Autodesk Fusion 360 part; units mm, degrees
(part 2 of 2)
  line L920 (94.2802, 13.415) -> (94.312, 13.3328)
  line L921 (90.8458, 12.0108) -> (90.0144, 12.5127)
  line L922 (98.4562, 13.1514) -> (98.2574, 14.132)
  line L923 (107.9148, 10.617) -> (107.3286, 10.4149)
  line L924 (98.2574, 14.132) -> (98.2624, 14.3913)
  line L925 (86.8526, 11.9567) -> (86.9805, 11.3055)
  line L926 (105.7225, 13.415) -> (105.8246, 13.9347)
  line L927 (107.3286, 10.4149) -> (105.3566, 11.5535)
  line L928 (94.1781, 13.9347) -> (94.2802, 13.415)
  line L929 (91.4254, 11.3668) -> (91.3001, 11.5939)
  line L930 (88.0455, 13.1497) -> (87.3969, 12.6054)
  line L931 (87.4895, 9.9878) -> (87.9914, 9.1564)
  line L932 (97.6083, 15.8299) -> (96.7216, 16.9295)
  line L933 (108.5772, 11.3668) -> (107.9148, 10.617)
  line L934 (94.6461, 11.5535) -> (92.674, 10.4149)
  line L935 (105.3566, 11.5535) -> (105.2385, 12.1621)
  line L936 (87.9914, 9.1564) -> (88.3397, 8.7574)
  line L937 (88.3397, 8.7574) -> (88.4083, 8.702)
  line L938 (102.3944, 15.8299) -> (101.9253, 14.9795)
  line L939 (105.2385, 12.1621) -> (105.5566, 13.1108)
  line L940 (105.5566, 13.1108) -> (105.6907, 13.3328)
  line L941 (103.781, 17.3659) -> (103.2811, 16.9295)
  line L942 (90.0144, 12.5127) -> (88.6967, 13.0217)
  line L943 (86.9805, 11.3055) -> (87.4895, 9.9878)
  line L944 (95.3877, 17.2189) -> (94.592, 16.9293)
  line L945 (108.7578, 11.6625) -> (108.7025, 11.5939)
  line L946 (87.3969, 12.6054) -> (86.8526, 11.9567)
  line L947 (101.9253, 14.9795) -> (101.7539, 14.4784)
  line L948 (101.5465, 13.1514) -> (101.1399, 12.6833)
  line L949 (94.592, 16.9293) -> (94.3773, 16.3014)
  line L950 (103.2811, 16.9295) -> (102.3944, 15.8299)
  line L951 (105.8246, 13.9347) -> (105.8435, 14.9057)
  line L952 (101.1399, 12.6833) -> (98.8628, 12.6833)
  line L953 (94.3773, 16.3014) -> (94.1592, 14.9057)
  line L954 (96.2216, 17.3659) -> (95.3877, 17.2189)
  line L955 (94.1592, 14.9057) -> (94.1781, 13.9347)
  line L956 (108.7025, 11.5939) -> (108.5772, 11.3668)
  line L957 (94.7641, 12.1621) -> (94.6461, 11.5535)
  line L958 (94.446, 13.1108) -> (94.7641, 12.1621)
  line L959 (92.0879, 10.617) -> (91.4254, 11.3668)
  line L960 (96.7216, 16.9295) -> (96.2216, 17.3659)
  line L961 (94.312, 13.3328) -> (94.446, 13.1108)
  line L962 (87.84, 5.238) -> (86.8914, 5.5562)
  line L963 (89.3852, 7.9143) -> (89.5873, 7.3281)
  line L964 (101.7403, 14.3913) -> (101.7453, 14.132)
  line L965 (86.6694, 5.6902) -> (86.5872, 5.7219)
  line L966 (109.9882, 12.5127) -> (109.1568, 12.0108)
  line L967 (86.8914, 5.5562) -> (86.6694, 5.6902)
  line L968 (98.8628, 12.6833) -> (98.4562, 13.1514)
  line L969 (91.3001, 11.5939) -> (91.2448, 11.6625)
  line L970 (104.6149, 17.2189) -> (103.781, 17.3659)
  line L971 (105.4106, 16.9293) -> (104.6149, 17.2189)
  line L972 (105.6254, 16.3014) -> (105.4106, 16.9293)
  line L973 (88.4083, 8.702) -> (88.6354, 8.5768)
  line L974 (88.6354, 8.5768) -> (89.3852, 7.9143)
  line L975 (101.7539, 14.4784) -> (101.7403, 14.3913)
  line L976 (89.5873, 7.3281) -> (88.4487, 5.3561)
  line L977 (86.5872, 5.7219) -> (86.0675, 5.8241)
  line L978 (85.0965, 5.8431) -> (83.7008, 5.625)
  line L979 (88.4487, 5.3561) -> (87.84, 5.238)
  line L980 (86.0675, 5.8241) -> (85.0965, 5.8431)
  line L981 (83.7008, 5.625) -> (83.0729, 5.4103)
  line L982 (83.0729, -5.4081) -> (83.7008, -5.6228)
  line L983 (87.3189, 1.1396) -> (87.3189, -1.1375)
  line L984 (82.6363, -3.7785) -> (82.7833, -4.6124)
  line L985 (85.8702, 1.745) -> (86.8508, 1.5462)
  line L986 (83.0727, -3.2785) -> (82.6363, -3.7785)
  line L987 (86.6694, -5.688) -> (86.8914, -5.554)
  line L988 (82.7833, 4.6146) -> (82.6363, 3.7807)
  line L989 (82.6363, 3.7807) -> (83.0727, 3.2807)
  line L990 (85.0227, 1.925) -> (85.5238, 1.7535)
  line L991 (86.8914, -5.554) -> (87.84, -5.2359)
  line L992 (85.5238, 1.7535) -> (85.6109, 1.74)
  line L993 (84.1723, 2.394) -> (85.0227, 1.925)
  line L994 (85.5238, -1.7513) -> (85.0227, -1.9227)
  line L995 (85.0227, -1.9227) -> (84.1723, -2.3918)
  line L996 (85.6109, -1.7379) -> (85.5238, -1.7513)
  line L997 (105.6254, -16.2992) -> (105.8435, -14.9035)
  line L998 (94.3773, -16.2992) -> (94.592, -16.9271)
  line L999 (83.0727, 3.2807) -> (84.1723, 2.394)
  line L1000 (88.4487, -5.3539) -> (89.5873, -7.326)
  line L1001 (85.0965, -5.841) -> (86.0675, -5.8219)
  line L1002 (88.3397, -8.7552) -> (87.9914, -9.1542)
  line L1003 (95.3877, -17.2167) -> (96.2216, -17.3637)
  line L1004 (84.1723, -2.3918) -> (83.0727, -3.2785)
  line L1005 (82.7833, -4.6124) -> (83.0729, -5.4081)
  line L1006 (85.6109, 1.74) -> (85.8702, 1.745)
  line L1007 (86.0675, -5.8219) -> (86.5872, -5.7198)
  line L1008 (86.8508, -1.5441) -> (85.8702, -1.7429)
  line L1009 (86.5872, -5.7198) -> (86.6694, -5.688)
  line L1010 (86.8508, 1.5462) -> (87.3189, 1.1396)
  line L1011 (83.0729, 5.4103) -> (82.7833, 4.6146)
  line L1012 (87.3189, -1.1375) -> (86.8508, -1.5441)
  line L1013 (83.7008, -5.6228) -> (85.0965, -5.841)
  line L1014 (105.8435, -14.9035) -> (105.8246, -13.9325)
  line L1015 (98.2624, -14.3891) -> (98.2574, -14.1298)
  line L1016 (105.5566, -13.1086) -> (105.2385, -12.16)
  line L1017 (104.6149, -17.2167) -> (105.4106, -16.9271)
  line L1018 (90.0144, -12.5106) -> (90.8458, -12.0087)
  line L1019 (105.2385, -12.16) -> (105.3566, -11.5513)
  line L1020 (85.8702, -1.7429) -> (85.6109, -1.7379)
  line L1021 (105.8246, -13.9325) -> (105.7225, -13.4128)
  line L1022 (94.7641, -12.16) -> (94.446, -13.1086)
  line L1023 (101.5465, -13.1492) -> (101.7453, -14.1298)
  line L1024 (105.6907, -13.3306) -> (105.5566, -13.1086)
  line L1025 (89.3852, -7.9121) -> (88.6354, -8.5746)
  line L1026 (88.4083, -8.6999) -> (88.3397, -8.7552)
  line L1027 (94.2802, -13.4128) -> (94.1781, -13.9325)
  line L1028 (101.7403, -14.3891) -> (101.7539, -14.4762)
  line L1029 (105.7225, -13.4128) -> (105.6907, -13.3306)
  line L1030 (90.8458, -12.0087) -> (91.2448, -11.6604)
  line L1031 (89.5873, -7.326) -> (89.3852, -7.9121)
  line L1032 (88.0455, -13.1475) -> (88.6967, -13.0195)
  line L1033 (88.6967, -13.0195) -> (90.0144, -12.5106)
  line L1034 (103.2811, -16.9273) -> (103.781, -17.3637)
  line L1035 (92.674, -10.4128) -> (94.6461, -11.5513)
  line L1036 (107.9148, -10.6149) -> (108.5772, -11.3647)
  line L1037 (94.1781, -13.9325) -> (94.1592, -14.9035)
  line L1038 (96.2216, -17.3637) -> (96.7216, -16.9273)
  line L1039 (88.6354, -8.5746) -> (88.4083, -8.6999)
  line L1040 (94.592, -16.9271) -> (95.3877, -17.2167)
  line L1041 (94.312, -13.3306) -> (94.2802, -13.4128)
  line L1042 (98.2488, -14.4762) -> (98.2624, -14.3891)
  line L1043 (103.781, -17.3637) -> (104.6149, -17.2167)
  line L1044 (87.84, -5.2359) -> (88.4487, -5.3539)
  line L1045 (94.446, -13.1086) -> (94.312, -13.3306)
  line L1046 (101.7539, -14.4762) -> (101.9253, -14.9773)
  line L1047 (113.0221, 11.3055) -> (113.1501, 11.9567)
  line L1048 (98.4562, -13.1492) -> (98.8628, -12.6811)
  line L1049 (111.6629, -8.7552) -> (111.5943, -8.6999)
  line L1050 (98.2574, -14.1298) -> (98.4562, -13.1492)
  line L1051 (94.6461, -11.5513) -> (94.7641, -12.16)
  line L1052 (92.0879, -10.6149) -> (92.674, -10.4128)
  line L1053 (111.9571, -13.1475) -> (112.6058, -12.6032)
  line L1054 (91.4254, -11.3647) -> (92.0879, -10.6149)
  line L1055 (98.8628, -12.6811) -> (101.1399, -12.6811)
  line L1056 (91.3001, -11.5917) -> (91.4254, -11.3647)
  line L1057 (87.4895, -9.9856) -> (86.9805, -11.3034)
  line L1058 (105.4106, -16.9271) -> (105.6254, -16.2992)
  line L1059 (87.3969, -12.6032) -> (88.0455, -13.1475)
  line L1060 (86.9805, -11.3034) -> (86.8526, -11.9545)
  line L1061 (108.7025, -11.5917) -> (108.7578, -11.6604)
  line L1062 (105.3566, -11.5513) -> (107.3286, -10.4128)
  line L1063 (107.3286, -10.4128) -> (107.9148, -10.6149)
  line L1064 (110.6175, -7.9121) -> (110.4154, -7.326)
  line L1065 (98.0774, -14.9773) -> (98.2488, -14.4762)
  line L1066 (115.8303, -2.3918) -> (114.9799, -1.9227)
  line L1067 (87.9914, -9.1542) -> (87.4895, -9.9856)
  line L1068 (114.3917, 1.74) -> (114.4788, 1.7535)
  line L1069 (94.1592, -14.9035) -> (94.3773, -16.2992)
  line L1070 (116.3018, -5.6228) -> (116.9297, -5.4081)
  line L1071 (116.9299, 3.2807) -> (117.3664, 3.7807)
  line L1072 (102.3944, -15.8277) -> (103.2811, -16.9273)
  line L1073 (97.6083, -15.8277) -> (98.0774, -14.9773)
  line L1074 (101.1399, -12.6811) -> (101.5465, -13.1492)
  line L1075 (114.9061, -5.841) -> (116.3018, -5.6228)
  line L1076 (111.5943, -8.6999) -> (111.3673, -8.5746)
  line L1077 (101.9253, -14.9773) -> (102.3944, -15.8277)
  line L1078 (108.5772, -11.3647) -> (108.7025, -11.5917)
  line L1079 (91.2448, -11.6604) -> (91.3001, -11.5917)
  line L1080 (101.7453, -14.1298) -> (101.7403, -14.3891)
  line L1081 (86.8526, -11.9545) -> (87.3969, -12.6032)
  line L1082 (112.1626, 5.238) -> (111.5539, 5.3561)
  line L1083 (116.3018, 5.625) -> (114.9061, 5.8431)
  line L1084 (112.0112, 9.1564) -> (112.5131, 9.9878)
  line L1085 (108.7578, -11.6604) -> (109.1568, -12.0087)
  line L1086 (114.9061, 5.8431) -> (113.9351, 5.8241)
  line L1087 (111.306, -13.0195) -> (111.9571, -13.1475)
  line L1088 (96.7216, -16.9273) -> (97.6083, -15.8277)
  line L1089 (109.1568, 12.0108) -> (108.7578, 11.6625)
  line L1090 (114.4788, -1.7513) -> (114.3917, -1.7379)
  line L1091 (111.5539, 5.3561) -> (110.4154, 7.3281)
  line L1092 (113.1501, 11.9567) -> (112.6058, 12.6054)
  line L1093 (112.6837, -1.1375) -> (112.6837, 1.1396)
  line L1094 (115.8303, 2.394) -> (116.9299, 3.2807)
  line L1095 (110.6175, 7.9143) -> (111.3673, 8.5768)
  line L1096 (113.4154, 5.7219) -> (113.3332, 5.6902)
  line L1097 (112.5131, 9.9878) -> (113.0221, 11.3055)
  line L1098 (113.4154, -5.7198) -> (113.9351, -5.8219)
  line L1099 (112.6058, 12.6054) -> (111.9571, 13.1497)
  line L1100 (114.1324, -1.7429) -> (113.1518, -1.5441)
  line L1101 (110.4154, 7.3281) -> (110.6175, 7.9143)
  line L1102 (113.1518, 1.5462) -> (114.1324, 1.745)
  line L1103 (110.4154, -7.326) -> (111.5539, -5.3539)
  line L1104 (114.4788, 1.7535) -> (114.9799, 1.925)
  line L1105 (112.6058, -12.6032) -> (113.1501, -11.9545)
  line L1106 (113.1501, -11.9545) -> (113.0221, -11.3034)
  line L1107 (113.1112, 5.5562) -> (112.1626, 5.238)
  line L1108 (113.0221, -11.3034) -> (112.5131, -9.9856)
  line L1109 (109.1568, -12.0087) -> (109.9882, -12.5106)
  line L1110 (111.6629, 8.7574) -> (112.0112, 9.1564)
  line L1111 (114.1324, 1.745) -> (114.3917, 1.74)
  line L1112 (111.3673, -8.5746) -> (110.6175, -7.9121)
  line L1113 (111.306, 13.0217) -> (109.9882, 12.5127)
  line L1114 (112.1626, -5.2359) -> (113.1112, -5.554)
  line L1115 (117.3664, -3.7785) -> (116.9299, -3.2785)
  line L1116 (116.9297, 5.4103) -> (116.3018, 5.625)
  line L1117 (113.9351, -5.8219) -> (114.9061, -5.841)
  line L1118 (113.1112, -5.554) -> (113.3332, -5.688)
  line L1119 (111.3673, 8.5768) -> (111.5943, 8.702)
  line L1120 (117.2193, -4.6124) -> (117.3664, -3.7785)
  line L1121 (113.3332, -5.688) -> (113.4154, -5.7198)
  line L1122 (109.9882, -12.5106) -> (111.306, -13.0195)
  line L1123 (113.9351, 5.8241) -> (113.4154, 5.7219)
  line L1124 (116.9297, -5.4081) -> (117.2193, -4.6124)
  line L1125 (114.3917, -1.7379) -> (114.1324, -1.7429)
  line L1126 (111.5539, -5.3539) -> (112.1626, -5.2359)
  line L1127 (113.1518, -1.5441) -> (112.6837, -1.1375)
  line L1128 (113.3332, 5.6902) -> (113.1112, 5.5562)
  line L1129 (112.5131, -9.9856) -> (112.0112, -9.1542)
  line L1130 (116.9299, -3.2785) -> (115.8303, -2.3918)
  line L1131 (111.9571, 13.1497) -> (111.306, 13.0217)
  line L1132 (117.2193, 4.6146) -> (116.9297, 5.4103)
  line L1133 (117.3664, 3.7807) -> (117.2193, 4.6146)
  line L1134 (114.9799, -1.9227) -> (114.4788, -1.7513)
  line L1135 (92.674, 10.4149) -> (92.0879, 10.617)
  line L1136 (98.2488, 14.4784) -> (98.0774, 14.9795)
  line L1137 (111.5943, 8.702) -> (111.6629, 8.7574)
  line L1138 (114.9799, 1.925) -> (115.8303, 2.394)
  line L1139 (112.6837, 1.1396) -> (113.1518, 1.5462)
  line L1140 (112.0112, -9.1542) -> (111.6629, -8.7552)
  circle A0 centre (0, 0) radius 4
  line L1141 (102.5, 5) -> (97.5, 5)
  line L1142 (97.5, 5) -> (97.5, -5)
  line L1143 (97.5, -5) -> (102.5, -5)
  line L1144 (102.5, -5) -> (102.5, 5)
  line L1145 (102.5, 5) -> (97.5, -5) construction
  line L1146 (97.5, 5) -> (102.5, -5) construction
  arc A1 (11.1765, 46.1664) -> (5, 41.3068) centre (10, 41.3068) ccw
  arc A2 (-5, 41.3068) -> (-11.1765, 46.1664) centre (-10, 41.3068) ccw
  arc A3 (-46.1664, 11.1765) -> (-41.3068, 5) centre (-41.3068, 10) ccw
  arc A4 (-41.3068, -5) -> (-46.1664, -11.1765) centre (-41.3068, -10) ccw
  arc A5 (-11.1765, -46.1664) -> (-5, -41.3068) centre (-10, -41.3068) ccw
  arc A6 (5, -41.3068) -> (11.1765, -46.1664) centre (10, -41.3068) ccw
  arc A7 (46.1664, -11.1765) -> (41.3068, -5) centre (41.3068, -10) ccw
  arc A8 (41.3068, 5) -> (46.1664, 11.1765) centre (41.3068, 10) ccw
  arc A9 (-11.1765, 46.1664) -> (-46.1664, 11.1765) centre (0, 0) ccw
  arc A10 (46.1664, 11.1765) -> (11.1765, 46.1664) centre (0, 0) ccw
  arc A11 (-46.1664, -11.1765) -> (-11.1765, -46.1664) centre (0, 0) ccw
  arc A12 (11.1765, -46.1664) -> (46.1664, -11.1765) centre (0, 0) ccw
  arc A13 (-18.3303, -5) -> (-5, -18.3303) centre (0, 0) ccw
  arc A14 (5, -18.3303) -> (18.3303, -5) centre (0, 0) ccw
  arc A15 (18.3303, 5) -> (5, 18.3303) centre (0, 0) ccw
  arc A16 (-5, 18.3303) -> (-18.3303, 5) centre (0, 0) ccw
  line L1147 (-5, 41.3068) -> (-5, 18.3303)
  line L1148 (-5, -18.3303) -> (-5, -41.3068)
  line L1149 (5, -41.3068) -> (5, -18.3303)
  line L1150 (5, 18.3303) -> (5, 41.3068)
  line L1151 (18.3303, 5) -> (41.3068, 5)
  line L1152 (41.3068, -5) -> (18.3303, -5)
  line L1153 (-18.3303, -5) -> (-41.3068, -5)
  line L1154 (-41.3068, 5) -> (-18.3303, 5)
  line L1155 (133.0727, 3.2807) -> (134.1723, 2.394)
  line L1156 (135.0227, 1.925) -> (135.5238, 1.7535)
  line L1157 (139.5873, 7.3281) -> (138.4487, 5.3561)
  line L1158 (136.6694, 5.6902) -> (136.5872, 5.7219)
  line L1159 (137.3969, 12.6054) -> (136.8526, 11.9567)
  line L1160 (148.4562, 13.1514) -> (148.2574, 14.132)
  line L1161 (138.0455, 13.1497) -> (137.3969, 12.6054)
  line L1162 (135.8702, 1.745) -> (136.8508, 1.5462)
  line L1163 (138.3397, 8.7574) -> (138.4083, 8.702)
  line L1164 (134.1723, 2.394) -> (135.0227, 1.925)
  line L1165 (136.8508, 1.5462) -> (137.3189, 1.1396)
  line L1166 (132.7833, 4.6146) -> (132.6363, 3.7807)
  line L1167 (138.6967, 13.0217) -> (138.0455, 13.1497)
  line L1168 (148.0774, 14.9795) -> (147.6083, 15.8299)
  line L1169 (138.4487, 5.3561) -> (137.84, 5.238)
  line L1170 (132.6363, 3.7807) -> (133.0727, 3.2807)
  line L1171 (138.6354, 8.5768) -> (139.3852, 7.9143)
  line L1172 (136.8526, 11.9567) -> (136.9805, 11.3055)
  line L1173 (136.8914, 5.5562) -> (136.6694, 5.6902)
  line L1174 (137.9914, 9.1564) -> (138.3397, 8.7574)
  line L1175 (136.9805, 11.3055) -> (137.4895, 9.9878)
  line L1176 (137.4895, 9.9878) -> (137.9914, 9.1564)
  line L1177 (133.0729, 5.4103) -> (132.7833, 4.6146)
  line L1178 (136.5872, 5.7219) -> (136.0675, 5.8241)
  line L1179 (135.6109, 1.74) -> (135.8702, 1.745)
  line L1180 (136.0675, 5.8241) -> (135.0965, 5.8431)
  line L1181 (137.84, 5.238) -> (136.8914, 5.5562)
  line L1182 (139.3852, 7.9143) -> (139.5873, 7.3281)
  line L1183 (135.5238, 1.7535) -> (135.6109, 1.74)
  line L1184 (133.7008, 5.625) -> (133.0729, 5.4103)
  line L1185 (135.0965, 5.8431) -> (133.7008, 5.625)
  line L1186 (138.4083, 8.702) -> (138.6354, 8.5768)
  line L1187 (140.0144, 12.5127) -> (138.6967, 13.0217)
  line L1188 (137.3189, 1.1396) -> (137.3189, -1.1375)
  line L1189 (151.5465, -13.1492) -> (151.7453, -14.1298)
  line L1190 (154.6149, -17.2167) -> (155.4106, -16.9271)
  line L1191 (151.9253, -14.9773) -> (152.3944, -15.8277)
  line L1192 (162.6058, -12.6032) -> (163.1501, -11.9545)
  line L1193 (158.7578, -11.6604) -> (159.1568, -12.0087)
  line L1194 (155.2385, -12.16) -> (155.3566, -11.5513)
  line L1195 (155.6254, -16.2992) -> (155.8435, -14.9035)
  line L1196 (158.5772, -11.3647) -> (158.7025, -11.5917)
  line L1197 (155.7225, -13.4128) -> (155.6907, -13.3306)
  line L1198 (159.1568, -12.0087) -> (159.9882, -12.5106)
  line L1199 (152.3944, -15.8277) -> (153.2811, -16.9273)
  line L1200 (158.7025, -11.5917) -> (158.7578, -11.6604)
  line L1201 (161.9571, -13.1475) -> (162.6058, -12.6032)
  line L1202 (161.306, -13.0195) -> (161.9571, -13.1475)
  line L1203 (167.3664, -3.7785) -> (166.9299, -3.2785)
  line L1204 (161.3673, -8.5746) -> (160.6175, -7.9121)
  line L1205 (151.7403, -14.3891) -> (151.7539, -14.4762)
  line L1206 (164.3917, -1.7379) -> (164.1324, -1.7429)
  line L1207 (163.1112, -5.554) -> (163.3332, -5.688)
  line L1208 (161.5943, -8.6999) -> (161.3673, -8.5746)
  line L1209 (155.5566, -13.1086) -> (155.2385, -12.16)
  line L1210 (165.8303, -2.3918) -> (164.9799, -1.9227)
  line L1211 (162.5131, -9.9856) -> (162.0112, -9.1542)
  line L1212 (151.1399, -12.6811) -> (151.5465, -13.1492)
  line L1213 (161.5539, -5.3539) -> (162.1626, -5.2359)
  line L1214 (166.9299, -3.2785) -> (165.8303, -2.3918)
  line L1215 (163.3332, -5.688) -> (163.4154, -5.7198)
  line L1216 (167.2193, -4.6124) -> (167.3663, -3.7785)
  line L1217 (157.9148, -10.6149) -> (158.5772, -11.3647)
  line L1218 (164.1324, -1.7429) -> (163.1518, -1.5441)
  line L1219 (163.9351, -5.8219) -> (164.9061, -5.841)
  line L1220 (166.3018, -5.6228) -> (166.9297, -5.4081)
  line L1221 (164.9799, -1.9227) -> (164.4788, -1.7513)
  line L1222 (162.1626, -5.2359) -> (163.1112, -5.554)
  line L1223 (160.4154, -7.326) -> (161.5539, -5.3539)
  line L1224 (166.9297, -5.4081) -> (167.2193, -4.6124)
  line L1225 (162.0112, -9.1542) -> (161.6629, -8.7552)
  line L1226 (163.4154, -5.7198) -> (163.9351, -5.8219)
  line L1227 (160.6175, -7.9121) -> (160.4154, -7.326)
  line L1228 (163.1518, -1.5441) -> (162.6837, -1.1375)
  line L1229 (164.4788, -1.7513) -> (164.3917, -1.7379)
  line L1230 (164.9061, -5.841) -> (166.3018, -5.6228)
  line L1231 (161.6629, -8.7552) -> (161.5943, -8.6999)
  line L1232 (161.5943, 8.702) -> (161.6629, 8.7574)
  line L1233 (166.9297, 5.4103) -> (166.3018, 5.625)
  line L1234 (164.4788, 1.7535) -> (164.9799, 1.925)
  line L1235 (163.1518, 1.5462) -> (164.1324, 1.745)
  line L1236 (164.9799, 1.925) -> (165.8303, 2.394)
  line L1237 (163.0221, -11.3034) -> (162.5131, -9.9856)
  line L1238 (161.6629, 8.7574) -> (162.0112, 9.1564)
  line L1239 (167.3664, 3.7807) -> (167.2193, 4.6146)
  line L1240 (162.0112, 9.1564) -> (162.5131, 9.9878)
  line L1241 (166.9299, 3.2807) -> (167.3663, 3.7807)
  line L1242 (167.2193, 4.6146) -> (166.9297, 5.4103)
  line L1243 (160.4154, 7.3281) -> (160.6175, 7.9143)
  line L1244 (164.9061, 5.8431) -> (163.9351, 5.8241)
  line L1245 (161.5539, 5.3561) -> (160.4154, 7.3281)
  line L1246 (151.7453, 14.132) -> (151.5465, 13.1514)
  line L1247 (163.0221, 11.3055) -> (163.1501, 11.9567)
  line L1248 (162.1626, 5.238) -> (161.5539, 5.3561)
  line L1249 (161.9571, 13.1497) -> (161.306, 13.0217)
  line L1250 (155.8435, 14.9057) -> (155.6254, 16.3014)
  line L1251 (151.7539, 14.4784) -> (151.7403, 14.3913)
  line L1252 (161.3673, 8.5768) -> (161.5943, 8.702)
  line L1253 (159.1568, 12.0108) -> (158.7578, 11.6625)
  line L1254 (151.5465, 13.1514) -> (151.1399, 12.6833)
  line L1255 (158.7578, 11.6625) -> (158.7025, 11.5939)
  line L1256 (155.4106, 16.9293) -> (154.6149, 17.2189)
  line L1257 (155.8246, 13.9347) -> (155.8435, 14.9057)
  line L1258 (160.6175, 7.9143) -> (161.3673, 8.5768)
  line L1259 (166.3018, 5.625) -> (164.9061, 5.8431)
  line L1260 (164.1324, 1.745) -> (164.3917, 1.74)
  line L1261 (162.5131, 9.9878) -> (163.0221, 11.3055)
  line L1262 (162.6058, 12.6054) -> (161.9571, 13.1497)
  line L1263 (155.6254, 16.3014) -> (155.4106, 16.9293)
  line L1264 (163.1112, 5.5562) -> (162.1626, 5.238)
  line L1265 (163.1501, 11.9567) -> (162.6058, 12.6054)
  line L1266 (152.3944, 15.8299) -> (151.9253, 14.9795)
  line L1267 (151.7403, 14.3913) -> (151.7453, 14.132)
  line L1268 (165.8303, 2.394) -> (166.9299, 3.2807)
  line L1269 (162.6837, 1.1396) -> (163.1518, 1.5462)
  line L1270 (164.3917, 1.74) -> (164.4788, 1.7535)
  line L1271 (163.3332, 5.6902) -> (163.1112, 5.5562)
  line L1272 (163.9351, 5.8241) -> (163.4154, 5.7219)
  line L1273 (163.4154, 5.7219) -> (163.3332, 5.6902)
  line L1274 (155.7225, 13.415) -> (155.8246, 13.9347)
  line L1275 (151.9253, 14.9795) -> (151.7539, 14.4784)
  line L1276 (147.6083, -15.8277) -> (148.0774, -14.9773)
  line L1277 (157.3286, 10.4149) -> (155.3566, 11.5535)
  line L1278 (155.2385, 12.1621) -> (155.5566, 13.1108)
  line L1279 (148.2488, -14.4762) -> (148.2624, -14.3891)
  line L1280 (144.592, -16.9271) -> (145.3877, -17.2167)
  line L1281 (144.7641, -12.16) -> (144.446, -13.1086)
  line L1282 (162.6837, -1.1375) -> (162.6837, 1.1396)
  line L1283 (153.2811, 16.9295) -> (152.3944, 15.8299)
  line L1284 (148.2574, -14.1298) -> (148.4562, -13.1492)
  line L1285 (155.3566, 11.5535) -> (155.2385, 12.1621)
  line L1286 (140.8458, -12.0087) -> (141.2448, -11.6604)
  line L1287 (142.674, -10.4128) -> (144.6461, -11.5513)
  line L1288 (146.7216, -16.9273) -> (147.6083, -15.8277)
  line L1289 (141.2448, -11.6604) -> (141.3001, -11.5917)
  line L1290 (158.5772, 11.3668) -> (157.9148, 10.617)
  line L1291 (154.6149, 17.2189) -> (153.781, 17.3659)
  line L1292 (161.306, 13.0217) -> (159.9882, 12.5127)
  line L1293 (144.1592, -14.9035) -> (144.3773, -16.2992)
  line L1294 (157.9148, 10.617) -> (157.3286, 10.4149)
  line L1295 (148.0774, -14.9773) -> (148.2488, -14.4762)
  line L1296 (141.3001, -11.5917) -> (141.4254, -11.3647)
  line L1297 (155.5566, 13.1108) -> (155.6907, 13.3328)
  line L1298 (158.7025, 11.5939) -> (158.5772, 11.3668)
  line L1299 (141.4254, -11.3647) -> (142.0879, -10.6149)
  line L1300 (153.781, 17.3659) -> (153.2811, 16.9295)
  line L1301 (142.0879, -10.6149) -> (142.674, -10.4128)
  line L1302 (159.9882, 12.5127) -> (159.1568, 12.0108)
  line L1303 (155.6907, 13.3328) -> (155.7225, 13.415)
  line L1304 (144.1781, -13.9325) -> (144.1592, -14.9035)
  line L1305 (140.0144, -12.5106) -> (140.8458, -12.0087)
  line L1306 (148.4562, -13.1492) -> (148.8628, -12.6811)
  line L1307 (144.312, -13.3306) -> (144.2802, -13.4128)
  line L1308 (144.2802, -13.4128) -> (144.1781, -13.9325)
  line L1309 (137.3189, -1.1375) -> (136.8508, -1.5441)
  line L1310 (134.1723, -2.3918) -> (133.0727, -3.2785)
  line L1311 (137.9914, -9.1542) -> (137.4895, -9.9856)
  line L1312 (135.0965, -5.841) -> (136.0675, -5.8219)
  line L1313 (136.8914, -5.554) -> (137.84, -5.2359)
  line L1314 (148.2624, -14.3891) -> (148.2574, -14.1298)
  line L1315 (138.3397, -8.7552) -> (137.9914, -9.1542)
  line L1316 (133.0729, -5.4081) -> (133.7008, -5.6228)
  line L1317 (137.3969, -12.6032) -> (138.0455, -13.1475)
  line L1318 (138.0455, -13.1475) -> (138.6967, -13.0195)
  line L1319 (144.446, -13.1086) -> (144.312, -13.3306)
  line L1320 (136.0675, -5.8219) -> (136.5872, -5.7198)
  line L1321 (138.6354, -8.5746) -> (138.4083, -8.6999)
  line L1322 (151.1399, 12.6833) -> (148.8628, 12.6833)
  line L1323 (144.3773, -16.2992) -> (144.592, -16.9271)
  line L1324 (138.4083, -8.6999) -> (138.3397, -8.7552)
  line L1325 (136.8526, -11.9545) -> (137.3969, -12.6032)
  line L1326 (144.6461, -11.5513) -> (144.7641, -12.16)
  line L1327 (136.9805, -11.3034) -> (136.8526, -11.9545)
  line L1328 (135.0227, -1.9227) -> (134.1723, -2.3918)
  line L1329 (136.5872, -5.7198) -> (136.6694, -5.688)
  line L1330 (139.5873, -7.326) -> (139.3852, -7.9121)
  line L1331 (139.3852, -7.9121) -> (138.6354, -8.5746)
  line L1332 (138.4487, -5.3539) -> (139.5873, -7.326)
  line L1333 (132.6363, -3.7785) -> (132.7833, -4.6124)
  line L1334 (133.0727, -3.2785) -> (132.6363, -3.7785)
  line L1335 (132.7833, -4.6124) -> (133.0729, -5.4081)
  line L1336 (146.2216, -17.3637) -> (146.7216, -16.9273)
  line L1337 (145.3877, -17.2167) -> (146.2216, -17.3637)
  line L1338 (137.4895, -9.9856) -> (136.9805, -11.3034)
  line L1339 (137.84, -5.2359) -> (138.4487, -5.3539)
  line L1340 (135.6109, -1.7379) -> (135.5238, -1.7513)
  line L1341 (135.5238, -1.7513) -> (135.0227, -1.9227)
  line L1342 (148.8628, -12.6811) -> (151.1399, -12.6811)
  line L1343 (147.6083, 15.8299) -> (146.7216, 16.9295)
  line L1344 (136.6694, -5.688) -> (136.8914, -5.554)
  line L1345 (144.592, 16.9293) -> (144.3773, 16.3014)
  line L1346 (148.2488, 14.4784) -> (148.0774, 14.9795)
  line L1347 (148.2624, 14.3913) -> (148.2488, 14.4784)
  line L1348 (144.1781, 13.9347) -> (144.2802, 13.415)
  line L1349 (141.3001, 11.5939) -> (141.2448, 11.6625)
  line L1350 (146.7216, 16.9295) -> (146.2216, 17.3659)
  line L1351 (142.674, 10.4149) -> (142.0879, 10.617)
  line L1352 (144.7641, 12.1621) -> (144.6461, 11.5535)
  line L1353 (142.0879, 10.617) -> (141.4254, 11.3668)
  line L1354 (133.7008, -5.6228) -> (135.0965, -5.841)
  line L1355 (141.4254, 11.3668) -> (141.3001, 11.5939)
  line L1356 (138.6967, -13.0195) -> (140.0144, -12.5106)
  line L1357 (144.312, 13.3328) -> (144.446, 13.1108)
  line L1358 (146.2216, 17.3659) -> (145.3877, 17.2189)
  line L1359 (141.2448, 11.6625) -> (140.8458, 12.0108)
  line L1360 (144.2802, 13.415) -> (144.312, 13.3328)
  line L1361 (144.446, 13.1108) -> (144.7641, 12.1621)
  line L1362 (144.3773, 16.3014) -> (144.1592, 14.9057)
  line L1363 (144.1592, 14.9057) -> (144.1781, 13.9347)
  line L1364 (140.8458, 12.0108) -> (140.0144, 12.5127)
  line L1365 (145.3877, 17.2189) -> (144.592, 16.9293)
  line L1366 (144.6461, 11.5535) -> (142.674, 10.4149)
  line L1367 (148.2574, 14.132) -> (148.2624, 14.3913)
  line L1368 (135.8702, -1.7429) -> (135.6109, -1.7379)
  line L1369 (136.8508, -1.5441) -> (135.8702, -1.7429)
  line L1370 (148.8628, 12.6833) -> (148.4562, 13.1514)
  line L1371 (157.3286, -10.4128) -> (157.9148, -10.6149)
  line L1372 (155.3566, -11.5513) -> (157.3286, -10.4128)
  line L1373 (151.7453, -14.1298) -> (151.7403, -14.3891)
  line L1374 (163.1501, -11.9545) -> (163.0221, -11.3034)
  line L1375 (153.2811, -16.9273) -> (153.781, -17.3637)
  line L1376 (153.781, -17.3637) -> (154.6149, -17.2167)
  line L1377 (155.6907, -13.3306) -> (155.5566, -13.1086)
  line L1378 (155.8246, -13.9325) -> (155.7225, -13.4128)
  line L1379 (155.8435, -14.9035) -> (155.8246, -13.9325)
  line L1380 (155.4106, -16.9271) -> (155.6254, -16.2992)
  line L1381 (159.9882, -12.5106) -> (161.306, -13.0195)
  line L1382 (151.7539, -14.4762) -> (151.9253, -14.9773)
  line L1383 (151.75, 2.5) -> (148.25, 2.5)
  line L1384 (148.25, 2.5) -> (148.25, -2.5)
  line L1385 (148.25, -2.5) -> (151.75, -2.5)
  line L1386 (151.75, -2.5) -> (151.75, 2.5)
  line L1387 (151.75, 2.5) -> (148.25, -2.5) construction
  line L1388 (148.25, 2.5) -> (151.75, -2.5) construction
  point P0 (100, 0)
  point P1 (150, 0)
  dimension "d1" = 95
  dimension "d2" = 8
  dimension "d3" = 38
  dimension "d8" = 10
  dimension "d11" = 10
  dimension "d16" = 10
  dimension "d17" = 5
  dimension "d20" = 3.5
  dimension "d21" = 5
  constraint concentric A0 A11
  constraint concentric A11 A15
  constraint parallel L1147 L1149
  constraint coincident A0.centre A9.centre
  constraint parallel L1152 L1154
  constraint horizontal L1154
  constraint tangent A1 A11
  constraint tangent A1 L1149
  constraint tangent A2 A11
  constraint tangent A2 L1147
  constraint perpendicular L1141 L1142
  constraint parallel L1141 L1143
  constraint parallel L1142 L1144
  constraint horizontal L1141
  constraint coincident L1145 P0
  constraint coincident L1146 P0
  constraint coincident A2.end A11
  constraint coincident A6.end A11
  constraint coincident A8.end A11
  constraint concentric A9 A11
  constraint concentric A10 A11
  constraint concentric A11 A12
  constraint coincident A13.start L1152
  constraint concentric A13 A15
  constraint coincident A15.start L1154
  constraint coincident A13.end L1147
  constraint concentric A13 A14
  constraint coincident A15.end L1149
  constraint concentric A15 A16
  constraint collinear L1147 L1148
  constraint collinear L1149 L1150
  constraint collinear L1151 L1154
  constraint perpendicular L1383 L1384
  constraint parallel L1383 L1385
  constraint parallel L1384 L1386
  constraint horizontal L1383
  constraint coincident L1387 P1
  constraint coincident L1388 P1
  measures "d1" diameter of A11
  measures "d2" diameter of A0
  measures "d3" diameter of A15
  measures "d8" diameter of A1
  measures "d11" diameter of A2
  measures "d16" distance of L1141.end L1142.end
  measures "d17" distance of L1142.end L1143.end
  measures "d20" distance of L1384.end L1385.end
  measures "d21" distance of L1383.end L1384.end
extrude "Extrude1" add sketch "Sketch1" along normal blind 6 contours L0 L1 L2 L3 L4 L5 L6 L7 L8 L9 L10 L11 L12 L13 L14 L15 L16 L17 L18 L19 L20 L21 L22 L23 L24 L25 L26 L27 L28 L29 L30 L31 L32 L33 L34 L35 L36 L37 L38 L39 L40 L41 L42 L43 L44 L45 L46 L47 L48 L49 L50 L51 L52 L53 L54 L55 L56 L57 L58 L59 L60 L61 L62 L63 L64 L65 L66 L67 L68 L69 L70 L71 L72 L73 L74 L75 L76 L77 L78 L79 L80 L81 L82 L83 L84 L85 L86 L87 L88 L89 L90 L91 L92 L93 L94 L95 L96 L97 L98 L99 L100 L101 L102 L103 L104 L105 L106 L107 L108 L109 L110 L111 L112 L113 L114 L115 L116 L117 L118 L119 L120 L121 L122 L123 L124 L125 L126 L127 L128 L129 L130 L131 L132 L133 L134 L135 L136 L137 L138 L139 L140 L141 L142 L143 L144 L145 L146 L147 L148 L149 L150 L151 L152 L153 L154 L155 L156 L157 L158 L159 L160 L161 L162 L163 L164 L165 L166 L167 L168 L169 L170 L171 L172 L173 L174 L175 L176 L177 L178 L179 L180 L181 L182 L183 L184 L185 L186 L187 L188 L189 L190 L191 L192 L193 L194 L195 L196 L197 L198 L199 L200 L201 L202 L203 L204 L205 L206 L207 L208 L209 L210 L211 L212 L213 L214 L215 L216 L217 L218 L219 L220 L221 L222 L223 L224 L225 L226 L227 L228 L229 L230 L231 L232 L233 L234 L235 L236 L237 L238 L239 L240 L241 L242 L243 L244 L245 L246 L247 L248 L249 L250 L251 L252 L253 L254 L255 L256 L257 L258 L259 L260 L261 L262 L263 L264 L265 L266 L267 L268 L269 L270 L271 L272 L273 L274 L275 L276 L277 L278 L279 L280 L281 L282 L283 L284 L285 L286 L287 L288 L289 L290 L291 L292 L293 L294 L295 L296 L297 L298 L299 L300 L301 L302 L303 L304 L305 L306 L307 L308 L309 L310 L311 L312 L313 L314 L315 L316 L317 L318 L319 L320 L321 L322 L323 L324 L325 L326 L327 L328 L329 L330 L331 L332 L333 L334 L335 L336 L337 L338 L339 L340 L341 L342 L343 L344 L345 L346 L347 L348 L349 L350 L351 L352 L353 L354 L355 L356 L357 L358 L359 L360 L361 L362 L363 L364 L365 L366 L367 L368 L369 L370 L371 L372 L373 L374 L375 L376 L377 L378 L379 L380 L381 L382 L383 L384 L385 L386 L387 L388 L389 L390 L391 L392 L393 L394 L395 L396 L397 L398 L399 L400 L401 L402 L403 L404 L405 L406 L407 L408 L409 L410 L411 L412 L413 L414 L415 L416 L417 L418 L419 L420 L421 L422 L423 L424 L425 L426 L427 L428 L429 L430 L431 L432 L433 L434 L435 L436 L437 L438 L439 L440 L441 L442 L443 L444 L445 L446 L447 L448 L449 L450 L451 L452 L453 L454 L455 L456 L457 L458 L459 L460 L461 L462 L463 L464 L465 L466 L467 L468 L469 L470 L471 L472 L473 L474 L475 L476 L477 L478 L479 L480 L481 L482 L483 L484 L485 L486 L487 L488 L489 L490 L491 L492 L493 L494 L495 L496 L497 L498 L499 L500 L501 L502 L503 L504 L505 L506 L507 L508 L509 L510 L511 L512 L513 L514 L515 L516 L517 L518 L519 L520 L521 L522 L523 L524 L525 L526 L527 L528 L529 L530 L531 L532 L533 L534 L535 L536 L537 L538 L539 L540 L541 L542 L543 L544 L545 L546 L547 L548 L549 L550 L551 L552 L553 L554 L555 L556 L557 L558 L559 L560 L561 L562 L563 L564 L565 L566 L567 L568 L569 L570 L571 L572 L573 L574 L575 L576 L577 L578 L579 L580 L581 L582 L583 L584 L585 L586 L587 L588 L589 L590 L591 L592 L593 L594 L595 L596 L597 L598 L599 L600 L601 L602 L603 L604 L605 L606 L607 L608 L609 L610 L611 L612 L613 L614 L615 L616 L617 L618 L619 L620 L621 L622 L623 L624 L625 L626 L627 L628 L629 L630 L631 L632 L633 L634 L635 L636 L637 L638 L639 L640 L641 L642 L643 L644 L645 L646 L647 L648 L649 L650 L651 L652 L653 L654 L655 L656 L657 L658 L659 L660 L661 L662 L663 L664 L665 L666 L667 L668 L669 L670 L671 L672 L673 L674 L675 L676 L677 L678 L679 L680 L681 L682 L683 L684 L685 L686 L687 L688 L689 L690 L691 L692 L693 L694 L695 L696 L697 L698 L699 L700 L701 L702 L703 L704 L705 L706 L707 L708 L709 L710 L711 L712 L713 L714 L715 L716 L717 L718 L719 L720 L721 L722 L723 L724 L725 L726 L727 L728 L729 L730 L731 L732 L733 L734 L735 L736 L737 L738 L739 L740 L741 L742 L743 L744 L745 L746 L747 L748 L749 L750 L751 L752 L753 L754 L755 L756 L757 L758 L759 L760 L761 L762 L763 L764 L765 L766 L767 L768 L769 L770 L771 L772 L773 L774 L775 L776 L777 L778 L779 L780 L781 L782 L783 L784 L785 L786 L787 L788 L789 L790 L791 L792 L793 L794 L795 L796 L797 L798 L799 L800 L801 L802 L803 L804 L805 L806 L807 L808 L809 L810 L811 L812 L813 L814 L815 L816 L817 L818 L819 L820 L821 L822 L823 L824 L825 L826 L827 L828 L829 L830 L831 L832 L833 L834 L835 L836 L837 L838 L839 L840 L841 L842 L843 L844 L845 L846 L847 L848 L849 L850 L851 L852 L853 L854 L855 L856 L857 L858 L859 L860 L861 L862 L863 L864 L865 L866 L867 L868 L869 L870 L871 L872 L873 L874 L875 L876 L877 L878 L879 L880 L881 L882 L883 L884 L885 L886 L887 L888 L889 L890 L891 L892 L893 L894 L895 L896 L897 L898 L899 L900 L901 L902 L903 L904 L905 L906 L908 L909 L910 L911 L912
sketch "Sketch2" plane through (0, 0, 0) normal (0, 0, 1) x (1, 0, 0)
  arc A0 (-45.9554, -11.5073) -> (-10.9655, -46.4973) centre (0.211, -0.3309) ccw
  arc A1 (5.211, -18.6612) -> (18.5413, -5.3309) centre (0.211, -0.3309) ccw
  line L0 (-4.789, 40.9759) -> (-4.789, 17.9994)
  arc A2 (5.211, -41.6376) -> (11.3874, -46.4973) centre (10.211, -41.6376) ccw
  arc A3 (-10.9655, -46.4973) -> (-4.789, -41.6376) centre (-9.789, -41.6376) ccw
  arc A4 (11.3874, -46.4973) -> (46.3774, -11.5073) centre (0.211, -0.3309) ccw
  arc A5 (18.5413, 4.6691) -> (5.211, 17.9994) centre (0.211, -0.3309) ccw
  arc A6 (46.3774, -11.5073) -> (41.5177, -5.3309) centre (41.5177, -10.3309) ccw
  line L1 (-18.1193, -5.3309) -> (-41.0958, -5.3309)
  arc A7 (-18.1193, -5.3309) -> (-4.789, -18.6612) centre (0.211, -0.3309) ccw
  arc A8 (-41.0958, -5.3309) -> (-45.9554, -11.5073) centre (-41.0958, -10.3309) ccw
  arc A9 (-4.789, 17.9994) -> (-18.1193, 4.6691) centre (0.211, -0.3309) ccw
  line L2 (-4.789, -18.6612) -> (-4.789, -41.6376)
  arc A10 (41.5177, 4.6691) -> (46.3774, 10.8456) centre (41.5177, 9.6691) ccw
  line L3 (-41.0958, 4.6691) -> (-18.1193, 4.6691)
  line L4 (18.5413, 4.6691) -> (41.5177, 4.6691)
  line L5 (5.211, -41.6376) -> (5.211, -18.6612)
  arc A11 (-45.9554, 10.8456) -> (-41.0958, 4.6691) centre (-41.0958, 9.6691) ccw
  line L6 (41.5177, -5.3309) -> (18.5413, -5.3309)
  arc A12 (-4.789, 40.9759) -> (-10.9655, 45.8355) centre (-9.789, 40.9759) ccw
  arc A13 (11.3874, 45.8355) -> (5.211, 40.9759) centre (10.211, 40.9759) ccw
  arc A14 (46.3774, 10.8456) -> (11.3874, 45.8355) centre (0.211, -0.3309) ccw
  line L7 (5.211, 17.9994) -> (5.211, 40.9759)
  circle A15 centre (0.211, -0.3309) radius 4
  arc A16 (-10.9655, 45.8355) -> (-45.9554, 10.8456) centre (0.211, -0.3309) ccw
  circle A17 centre (0.211, -0.3309) radius 67.5
  point P0 (0.211, -0.3309)
  point P1 (0.211, -0.3309)
  dimension "d22" = 95
  dimension "d23" = 8
  dimension "d24" = 38
  dimension "d25" = 10
  dimension "d26" = 135
  constraint concentric A0 A15
  constraint concentric A0 A5
  constraint parallel L0 L5
  constraint coincident P1 P0
  constraint parallel L3 L6
  constraint horizontal L3
  constraint coincident A12.end A0
  constraint coincident A2.end A0
  constraint coincident A10.end A0
  constraint concentric A0 A16
  constraint concentric A0 A14
  constraint concentric A0 A4
  constraint coincident L1.start L6
  constraint concentric A5 A7
  constraint coincident A5.start L3
  constraint coincident A7.end L0
  constraint concentric A1 A7
  constraint coincident A5.end L5
  constraint concentric A5 A9
  constraint collinear L0 L2
  constraint collinear L5 L7
  constraint collinear L3 L4
  constraint concentric A15 A17
  measures "d22" diameter of A0
  measures "d23" diameter of A15
  measures "d24" diameter of A5
  measures "d25" diameter of A13
  measures "d26" diameter of A17
hidden bodies 1
